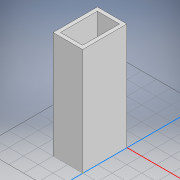
# Autodesk Inventor part: брус
Saved by Autodesk Inventor 2022 (Build 260153000, 153)
## iProperties
Created: 2022-05-16
Part Number: брус
Material: Типовые
Document SubType Name: Modeling
Designer: user
Density: 1 g/cm^3
Appearance: По умолчанию
Author: user
Autodesk Inventor part; units mm, degrees
ref_plane "YZ Plane" through (0, 0, 0) normal (1, 0, 0) x (0, 1, 0)
ref_plane "XZ Plane" through (0, 0, 0) normal (0, 1, 0) x (-1, 0, 0)
ref_plane "XY Plane" through (0, 0, 0) normal (0, 0, 1) x (1, 0, 0)
sketch "Эскиз1" plane through (0, 0, 0) normal (0, 1, 0) x (-1, 0, 0)
  line L0 (0, 0) -> (40, 0)
  line L1 (40, 0) -> (40, 60)
  line L2 (40, 60) -> (0, 60)
  line L3 (0, 60) -> (0, 0)
  dimension "d0" = 60
  dimension "d1" = 40
  constraints: 8 end point, 2 parallel, 1 horizontal, 1 perpendicular
  measures "d0" distance of L0.end L1.end
  measures "d1" distance of L0.start L0.end
extrude "Выдавливание1" add sketch "Эскиз1" along normal blind 190
sketch "Эскиз2" plane through (0, 190, 0) normal (0, 1, 0) x (1, 0, 0)
  line L0 (-35, -5) -> (-5, -5)
  line L1 (-5, -5) -> (-5, -55)
  line L2 (-5, -55) -> (-35, -55)
  line L3 (-35, -55) -> (-35, -5)
  line L4 (-40, 0) -> (-40, -60) projected
  line L5 (0, -60) -> (0, 0) projected
  line L6 (0, 0) -> (-40, 0) projected
  line L7 (-40, -60) -> (0, -60) projected
  dimension "d4" = 5
  dimension "d5" = 5
  dimension "d6" = 5
  dimension "d7" = 5
  constraints: 8 end point, 2 parallel, 1 horizontal, 1 perpendicular
  measures "d4" distance between parallel lines of L4 L3
  measures "d5" distance between parallel lines of L5 L1
  measures "d6" distance between parallel lines of L6 L0
  measures "d7" distance between parallel lines of L7 L2
extrude "Выдавливание2" cut sketch "Эскиз2" against normal through all contours L0 L1 L2 L3
sketch "Эскиз3" plane through (-40, 0, 60) normal (0, 0, 1) x (1, 0, 0)
  point P0 (40, 0)
sketch "Эскиз5" plane through (0, 190, 0) normal (0, 1, 0) x (1, 0, 0)
  line L0 (-5, -5) -> (-5, -55) projected
  line L1 (-5, -55) -> (-35, -55) projected
  line L2 (-35, -55) -> (-35, -5) projected
  line L3 (-35, -5) -> (-5, -5) projected
  line L4 (-40, 0) -> (-40, -60) projected
  line L5 (-40, -60) -> (0, -60) projected
  line L6 (0, -60) -> (0, 0) projected
  line L7 (0, 0) -> (-40, 0) projected
extrude "Выдавливание4" cut sketch "Эскиз5" against normal blind 45
equation "\"d5\" = d4"
equation "\"d6\" = d4"
equation "\"d7\" = d4"
